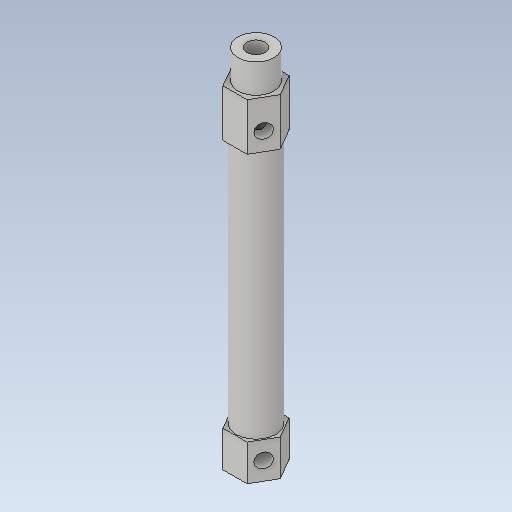
# Autodesk Inventor part: SMC_CJ1KB10-45(本体)
Saved by Autodesk Inventor 2020 (Build 240168000, 168)
## iProperties
Created: 2018-04-28
Part Number: SMC_CJ1KB10-45(本体)
Material: 一般
Document SubType Name: Modeling
Designer: Take
Density: 1 g/cm^3
Appearance: 既定
Author: Take
Autodesk Inventor part; units mm, degrees
ref_plane "YZ Plane" through (0, 0, 0) normal (1, 0, 0) x (0, 1, 0)
ref_plane "XZ Plane" through (0, 0, 0) normal (0, 1, 0) x (-1, 0, 0)
ref_plane "XY Plane" through (0, 0, 0) normal (0, 0, 1) x (1, 0, 0)
sketch "スケッチ1" plane through (0, 0, 0) normal (0, 1, 0) x (-1, 0, 0)
  line L0 (6.7, 0) -> (3.35, -5.8024)
  line L1 (3.35, -5.8024) -> (-3.35, -5.8024)
  line L2 (-3.35, -5.8024) -> (-6.7, 0)
  line L3 (-6.7, 0) -> (-3.35, 5.8024)
  line L4 (-3.35, 5.8024) -> (3.35, 5.8024)
  line L5 (3.35, 5.8024) -> (6.7, 0)
  point P0 (0, 0)
  point P1 (0, 0)
  dimension "d0" = 6.7
  constraints: 12 end point, 1 coincident, 13 other
  measures "d0" distance of L0.start point (0, 0)
extrude "押し出し1" add sketch "スケッチ1" along normal blind 10
sketch "スケッチ2" plane through (0, 10, 0) normal (0, 1, 0) x (1, 0, 0)
  circle A0 centre (0, 0) radius 5.5
  dimension "d3" = 11
  constraints: 1 centre point, 1 coincident
  measures "d3" diameter of A0
extrude "押し出し2" add sketch "スケッチ2" along normal blind 69
sketch "スケッチ3" plane through (0, 79, 0) normal (0, 1, 0) x (1, 0, 0)
  line L0 (-6.7, 0) -> (-3.35, 5.8024)
  line L1 (-3.35, 5.8024) -> (3.35, 5.8024)
  line L2 (3.35, 5.8024) -> (6.7, 0)
  line L3 (6.7, 0) -> (3.35, -5.8024)
  line L4 (3.35, -5.8024) -> (-3.35, -5.8024)
  line L5 (-3.35, -5.8024) -> (-6.7, 0)
  point P0 (0, 0)
  point P1 (0, 0)
  constraints: 12 end point, 1 coincident, 13 other
extrude "押し出し3" add sketch "スケッチ3" along normal blind 13.1
sketch "スケッチ4" plane through (0, 92.1, 0) normal (0, 1, 0) x (1, 0, 0)
  circle A0 centre (0, 0) radius 5
  dimension "d8" = 10
  constraints: 1 centre point, 1 coincident
  measures "d8" diameter of A0
extrude "押し出し4" add sketch "スケッチ4" along normal blind 8
sketch "スケッチ5" plane through (0, 100.1, 0) normal (0, 1, 0) x (1, 0, 0)
  circle A0 centre (0, 0) radius 2.5
  dimension "d11" = 5
  constraints: 1 centre point, 1 coincident
  measures "d11" diameter of A0
extrude "押し出し5" cut sketch "スケッチ5" against normal blind 50
sketch "スケッチ6" plane through (6.7, 0, 0) normal (0.866, 0, 0.5) x (0.5, 0, -0.866)
  line L0 (-3.35, 0) -> (-3.35, 10)
  line L1 (-8.85, 10) -> (2.15, 10) projected
  point P0 (-3.35, 5)
  constraints: 2 end point, 2 midpoint
hole "穴1" at (5.025, 5, 2.9012) direction (-0.866, 0, -0.5) diameter 4 depth 8.5
sketch "スケッチ7" plane through (6.7, 79, 0) normal (0.866, 0, 0.5) x (0.5, 0, -0.866)
  line L0 (0, 0) -> (-6.7, 0) projected
  line L1 (-3.35, 0) -> (-3.35, 13.1)
  line L2 (-6.7, 13.1) -> (0, 13.1) projected
  point P0 (-3.35, -79)
  point P1 (-3.35, 5)
  dimension "d21" = 5
  constraints: 2 end point, 2 midpoint, 1 point on line
  measures "d21" distance from line of point (-3.35, 5) L0
hole "穴2" at (5.025, 84, 2.9012) direction (-0.866, 0, -0.5) diameter 4 depth 5
